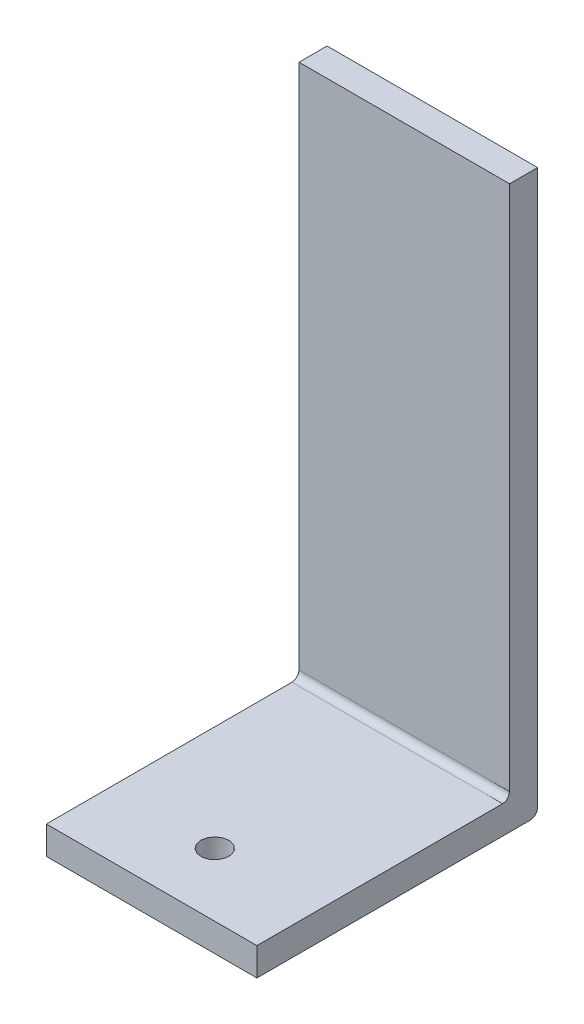
# Autodesk Inventor part: kątownik_bloczek
Saved by Autodesk Inventor 2014 (Build 180170000, 170)
## iProperties
Created: 2013-12-27
Part Number: kątownik_bloczek
Material: Ogólny
Document SubType Name: Modeling
Designer: Kuba
Density: 1 g/cm^3
Appearance: Domyślna
Author: Kuba
Autodesk Inventor part; units mm, degrees
ref_plane "YZ Plane" through (0, 0, 0) normal (1, 0, 0) x (0, 1, 0)
ref_plane "XZ Plane" through (0, 0, 0) normal (0, 1, 0) x (-1, 0, 0)
ref_plane "XY Plane" through (0, 0, 0) normal (0, 0, 1) x (1, 0, 0)
sketch "Szkic2" plane through (0, 0, 0) normal (1, 0, 0) x (0, 1, 0)
  line L0 (-10.1243, 0) -> (60.0207, 0)
  line L1 (0, -10.1243) -> (0, 60.0207)
  line L2 (0, 20) -> (0, 0.5)
  line L3 (0.5, 0) -> (40, 0)
  line L4 (40, 2) -> (2.5, 2)
  line L5 (2, 2.5) -> (2, 20)
  line L6 (2, 20) -> (0, 20)
  line L7 (40, 0) -> (40, 2)
  arc A0 (2, 2.5) -> (2.5, 2) centre (2.5, 2.5) ccw
  arc A1 (0, 0.5) -> (0.5, 0) centre (0.5, 0.5) ccw
  point P0 (0, 0)
  point P1 (0, 0)
  dimension "d4" = 2
  dimension "d5" = 2
  dimension "d6" = 40
  dimension "d7" = 20
  dimension "d8" = 0.5
  constraints: 16 end point, 4 point on circle, 4 point on line, 4 tangent, 2 centre point, 2 parallel, 2 perpendicular, 1 collinear, 1 equal radius
  measures "d4" distance between parallel lines of L5 L2
  measures "d5" distance between parallel lines of L0 L4
  measures "d6" distance between parallel lines of L1 L7
  measures "d7" distance between parallel lines of L0 L6
  measures "d8" radius of A0
extrude "Wyciągnięcie proste1" add sketch "Szkic2" along normal blind 15 contours A1 L1 L6 L5 A0 L4 L7 L0
sketch "Szkic3" plane through (0, 0, 0.5) normal (0, -1, 0) x (1, 0, 0)
  circle A0 centre (7.5, 15) radius 1
  point P0 (0, -0.5)
  dimension "d11" = 2
  constraints: 1 centre point
  measures "d11" diameter of A0
hole "Otwór1" at (7.5, 0, 15.5) direction (0, 1, 0) diameter 2 end through all
